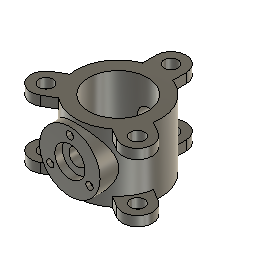
practice 2_ (Autodesk Fusion 360 design; units mm, degrees)
part number: 2026-06-02-19-11-36-206
Autodesk Fusion 360 part; units mm, degrees
sketch "Sketch1" plane through (0, 0, 0) normal (0, 0, 1) x (1, 0, 0)
  circle A0 centre (0, 0) radius 97
  circle A1 centre (0, 0) radius 140
  dimension "d1" = 194
  dimension "d2" = 280
  constraint coincident A0.centre A1.centre
  measures "d1" diameter of A0
  measures "d2" diameter of A1
extrude "Extrude1" add sketch "Sketch1" along normal blind 225
sketch "Sketch2" plane through (0, 0, 225) normal (0, 0, 1) x (-1, 0, 0)
  circle A0 centre (0, 0) radius 97
  circle A1 centre (0, 0) radius 140
  circle A2 centre (0, 0) radius 175 construction
  line L0 (0, 0) -> (0, -231.0128) construction
  circle A3 centre (0, -175) radius 23.5
  line L1 (50, -175) -> (50, -130.767)
  line L2 (-50, -175) -> (-50, -130.767)
  arc A4 (-49.4872, -167.8571) -> (49.4872, -167.8571) centre (0, -175) ccw
  dimension "d5" = 350
  dimension "d6" = 47
  dimension "d7" = 100
  constraint coincident A0.centre A1.centre
  constraint vertical L0
  constraint coincident A2 A3.centre
  constraint coincident L0 A3.centre
  constraint concentric A3 A4
  constraint coincident L1.start A4
  constraint tangent L1 A4
  constraint coincident L2.start A4
  constraint tangent L2 A4
  constraint parallel L1 L2
  constraint coincident A2 A4.end
  constraint coincident A2 A4.start
  constraint coincident A1 L2.end
  constraint coincident A1 L1.end
  measures "d5" diameter of A2
  measures "d6" diameter of A3
  measures "d7" diameter of A4
extrude "Extrude2" add sketch "Sketch2" against normal blind 32 contours A1 L1 L2 A4
pattern_circular "C-Pattern1" count 3 over 360 about axis through (0, 0, 1.75) along (0, 0, 1) of "Extrude2"
ref_plane "WorkPlane1" through (0, 22.331, 112.5) normal (0, 0, 1) x (1, 0, 0)
mirror "Mirror1" about plane through (0, 22.331, 112.5) normal (0, 0, 1) of "Extrude2", "C-Pattern1"
ref_plane "WorkPlane5" through (0, -160, 0) normal (0, 1, 0) x (0, 0, 1)
sketch "Sketch6" plane through (0, -160, 0) normal (0, 1, 0) x (1, 0, 0)
  circle A0 centre (0, -112.5) radius 100
  line L0 (-88.2475, 0) -> (88.2475, 0)
  dimension "d19" = 200
  dimension "d20" = 112.5
  constraint vertical origin A0.centre
  measures "d19" diameter of A0
  measures "d20" distance of A0.centre L0
extrude "Extrude3" add sketch "Sketch6" along normal up to surface end surface at (-37.048, 135.0091, 139.3333)
sketch "Sketch7" plane through (0, -160, 0) normal (0, -1, 0) x (1, 0, 0)
  circle A0 centre (0, 112.5) radius 100
  circle A1 centre (0, 112.5) radius 50
  circle A2 centre (0, 112.5) radius 28
  dimension "d23" = 100
  dimension "d24" = 56
  constraint concentric A0 A1
  constraint concentric A1 A2
  measures "d23" diameter of A1
  measures "d24" diameter of A2
extrude "Extrude4" cut sketch "Sketch7" against normal blind 25 contours A1
extrude "Extrude5" cut 1 faces at (5.8192, -160, 119.7971) along direction (0, 1, 0) through all
sketch "Sketch8" plane through (0, -160, 0) normal (0, -1, 0) x (1, 0, 0)
  circle A0 centre (0, 112.5) radius 100
  circle A1 centre (0, 112.5) radius 50
  circle A2 centre (0, 112.5) radius 75 construction
  circle A3 centre (0, 187.5) radius 12
  dimension "d28" = 150
  dimension "d29" = 24
  constraint concentric A0 A2
  constraint coincident A2 A3.centre
  constraint vertical A0.centre A3.centre
  measures "d28" diameter of A2
  measures "d29" diameter of A3
extrude "Extrude6" cut sketch "Sketch8" against normal blind 15 contours A3
pattern_circular "C-Pattern2" count 3 over 360 about axis through (0, -160, 112.5) along (0, 1, 0) of "Extrude6"
equation "d20 = ( 225 / 2 ) * 1 mm"
